Autodesk Inventor part; units mm, degrees
(part 2 of 2)
sketch "Sketch4" plane through (0, 0, 0.5) normal (0, 0, 1) x (1, 0, 0)
  line L0 (210, -1.9975) -> (0, -1.9975) projected
  line L1 (1.9975, -19.0025) -> (23.0025, -19.0025)
  line L2 (23.0025, -19.0025) -> (23.0025, -1.9975)
  line L3 (23.0025, -1.9975) -> (1.9975, -1.9975)
  line L4 (1.9975, -1.9975) -> (1.9975, -19.0025)
  line L5 (34.9975, -1.9975) -> (152.0025, -1.9975)
  line L6 (152.0025, -1.9975) -> (152.0025, -19.0025)
  line L7 (152.0025, -19.0025) -> (34.9975, -19.0025)
  line L8 (34.9975, -19.0025) -> (34.9975, -1.9975)
  line L9 (210, -24.25) -> (210, -1.9975) projected
  line L10 (163.4975, -1.9975) -> (210, -1.9975)
  line L11 (210, -1.9975) -> (210, -19.0025)
  line L12 (210, -19.0025) -> (163.4975, -19.0025)
  line L13 (163.4975, -19.0025) -> (163.4975, -1.9975)
  line L14 (200.5, -48.05) -> (200.5, -24.25) projected
  line L15 (200.5, -29.4975) -> (0, -29.4975)
  line L16 (0, -29.4975) -> (0, -122.9025)
  line L17 (0, -122.9025) -> (216.3009, -122.9025) projected
  line L18 (0, -122.9025) -> (216.3009, -122.9025)
  line L19 (216.3009, -122.9025) -> (216.3009, -105.3171)
  line L20 (216.3009, -103.8025) -> (205.25, -103.8025) projected
  line L21 (216.3009, -105.3171) -> (216.3009, -103.8025)
  line L22 (216.3009, -103.8025) -> (205.25, -103.8025)
  line L23 (200.5, -29.4975) -> (200.5, -48.05)
  line L24 (210.25, -67.15) -> (210.25, -48.05) projected
  line L25 (200.5, -48.05) -> (210.25, -48.05)
  line L26 (215, -67.15) -> (210.25, -67.15) projected
  line L27 (210.25, -48.05) -> (210.25, -67.15)
  line L28 (215, -86.25) -> (215, -67.15) projected
  line L29 (210.25, -67.15) -> (215, -67.15)
  line L30 (215, -67.15) -> (215, -86.25)
  line L31 (205.25, -103.8025) -> (205.25, -86.25) projected
  line L32 (215, -86.25) -> (205.25, -86.25)
  line L33 (205.25, -86.25) -> (205.25, -103.8025)
  line L34 (205.25, -103.8025) -> (216.3009, -103.8025)
  line L35 (163.4975, -1.9975) -> (210, -1.9975)
  line L36 (210, -1.9975) -> (210, -19.0025)
  line L37 (152.0025, -1.9975) -> (34.9975, -1.9975)
  line L38 (23.0025, -1.9975) -> (1.9975, -1.9975)
  line L39 (216.3009, -103.8025) -> (205.25, -103.8025) projected
  line L40 (205.25, -103.8025) -> (205.25, -86.25) projected
  line L41 (205.25, -86.25) -> (215, -86.25) projected
  line L42 (215, -86.25) -> (215, -67.15) projected
  line L43 (215, -67.15) -> (210.25, -67.15) projected
  line L44 (210.25, -67.15) -> (210.25, -48.05) projected
  line L45 (210.25, -48.05) -> (200.5, -48.05) projected
  line L46 (200.5, -48.05) -> (200.5, -24.25) projected
  line L47 (200.5, -24.25) -> (210, -24.25) projected
  line L48 (210, -24.25) -> (210, -1.9975) projected
  line L49 (210, -1.9975) -> (0, -1.9975) projected
  line L50 (0, -1.9975) -> (0, -122.9025) projected
  line L51 (0, -122.9025) -> (216.3009, -122.9025) projected
  line L52 (216.3009, -122.9025) -> (216.3009, -103.8025) projected
  line L53 (119.75, -21.25) -> (163.5, -21.25) projected
  line L54 (163.5, -21.25) -> (163.5, -28.75) projected
  line L55 (163.5, -28.75) -> (119.75, -28.75) projected
  line L56 (119.75, -28.75) -> (119.75, -21.25) projected
  line L57 (67.1017, -107.9725) -> (73.1018, -107.9725) projected
  line L58 (73.1018, -107.9725) -> (73.1018, -120.1725) projected
  line L59 (73.1018, -120.1725) -> (67.1017, -120.1725) projected
  line L60 (67.1017, -120.1725) -> (67.1017, -107.9725) projected
  line L61 (200.6018, -107.9725) -> (206.6018, -107.9725) projected
  line L62 (206.6018, -107.9725) -> (206.6018, -120.1725) projected
  line L63 (206.6018, -120.1725) -> (200.6018, -120.1725) projected
  line L64 (200.6018, -120.1725) -> (200.6018, -107.9725) projected
  line L65 (29, -50.5975) -> (35, -50.5975) projected
  line L66 (35, -50.5975) -> (35, -62.7975) projected
  line L67 (35, -62.7975) -> (29, -62.7975) projected
  line L68 (29, -62.7975) -> (29, -50.5975) projected
  line L69 (5, -50.5975) -> (11, -50.5975) projected
  line L70 (11, -50.5975) -> (11, -62.7975) projected
  line L71 (11, -62.7975) -> (5, -62.7975) projected
  line L72 (5, -62.7975) -> (5, -50.5975) projected
  line L73 (40.4975, -107.8975) -> (54.5025, -107.8975) projected
  line L74 (54.5025, -107.8975) -> (54.5025, -121.9025) projected
  line L75 (54.5025, -121.9025) -> (40.4975, -121.9025) projected
  line L76 (40.4975, -121.9025) -> (40.4975, -107.8975) projected
  line L77 (15.9975, -107.8975) -> (30.0025, -107.8975) projected
  line L78 (30.0025, -107.8975) -> (30.0025, -121.9025) projected
  line L79 (30.0025, -121.9025) -> (15.9975, -121.9025) projected
  line L80 (15.9975, -121.9025) -> (15.9975, -107.8975) projected
  line L81 (188.7475, -88.7975) -> (202.7525, -88.7975) projected
  line L82 (202.7525, -88.7975) -> (202.7525, -102.8025) projected
  line L83 (202.7525, -102.8025) -> (188.7475, -102.8025) projected
  line L84 (188.7475, -102.8025) -> (188.7475, -88.7975) projected
  line L85 (169.7475, -88.7975) -> (183.7525, -88.7975) projected
  line L86 (183.7525, -88.7975) -> (183.7525, -102.8025) projected
  line L87 (183.7525, -102.8025) -> (169.7475, -102.8025) projected
  line L88 (169.7475, -102.8025) -> (169.7475, -88.7975) projected
  line L89 (150.7475, -88.7975) -> (164.7525, -88.7975) projected
  line L90 (164.7525, -88.7975) -> (164.7525, -102.8025) projected
  line L91 (164.7525, -102.8025) -> (150.7475, -102.8025) projected
  line L92 (150.7475, -102.8025) -> (150.7475, -88.7975) projected
  line L93 (131.7475, -88.7975) -> (145.7525, -88.7975) projected
  line L94 (145.7525, -88.7975) -> (145.7525, -102.8025) projected
  line L95 (145.7525, -102.8025) -> (131.7475, -102.8025) projected
  line L96 (131.7475, -102.8025) -> (131.7475, -88.7975) projected
  line L97 (112.7475, -88.7975) -> (126.7525, -88.7975) projected
  line L98 (126.7525, -88.7975) -> (126.7525, -102.8025) projected
  line L99 (126.7525, -102.8025) -> (112.7475, -102.8025) projected
  line L100 (112.7475, -102.8025) -> (112.7475, -88.7975) projected
  line L101 (93.7475, -88.7975) -> (107.7525, -88.7975) projected
  line L102 (107.7525, -88.7975) -> (107.7525, -102.8025) projected
  line L103 (107.7525, -102.8025) -> (93.7475, -102.8025) projected
  line L104 (93.7475, -102.8025) -> (93.7475, -88.7975) projected
  line L105 (74.7475, -88.7975) -> (88.7525, -88.7975) projected
  line L106 (88.7525, -88.7975) -> (88.7525, -102.8025) projected
  line L107 (88.7525, -102.8025) -> (74.7475, -102.8025) projected
  line L108 (74.7475, -102.8025) -> (74.7475, -88.7975) projected
  line L109 (55.7475, -88.7975) -> (69.7525, -88.7975) projected
  line L110 (69.7525, -88.7975) -> (69.7525, -102.8025) projected
  line L111 (69.7525, -102.8025) -> (55.7475, -102.8025) projected
  line L112 (55.7475, -102.8025) -> (55.7475, -88.7975) projected
  line L113 (36.7475, -88.7975) -> (50.7525, -88.7975) projected
  line L114 (50.7525, -88.7975) -> (50.7525, -102.8025) projected
  line L115 (50.7525, -102.8025) -> (36.7475, -102.8025) projected
  line L116 (36.7475, -102.8025) -> (36.7475, -88.7975) projected
  line L117 (10.4975, -88.7975) -> (24.5025, -88.7975) projected
  line L118 (24.5025, -88.7975) -> (24.5025, -102.8025) projected
  line L119 (24.5025, -102.8025) -> (10.4975, -102.8025) projected
  line L120 (10.4975, -102.8025) -> (10.4975, -88.7975) projected
  line L121 (5.9975, -69.6975) -> (20.0025, -69.6975) projected
  line L122 (20.0025, -69.6975) -> (20.0025, -83.7025) projected
  line L123 (20.0025, -83.7025) -> (5.9975, -83.7025) projected
  line L124 (5.9975, -83.7025) -> (5.9975, -69.6975) projected
  line L125 (27.4975, -69.6975) -> (41.5025, -69.6975) projected
  line L126 (41.5025, -69.6975) -> (41.5025, -83.7025) projected
  line L127 (41.5025, -83.7025) -> (27.4975, -83.7025) projected
  line L128 (27.4975, -83.7025) -> (27.4975, -69.6975) projected
  line L129 (46.4975, -69.6975) -> (60.5025, -69.6975) projected
  line L130 (60.5025, -69.6975) -> (60.5025, -83.7025) projected
  line L131 (60.5025, -83.7025) -> (46.4975, -83.7025) projected
  line L132 (46.4975, -83.7025) -> (46.4975, -69.6975) projected
  line L133 (65.4975, -69.6975) -> (79.5025, -69.6975) projected
  line L134 (79.5025, -69.6975) -> (79.5025, -83.7025) projected
  line L135 (79.5025, -83.7025) -> (65.4975, -83.7025) projected
  line L136 (65.4975, -83.7025) -> (65.4975, -69.6975) projected
  line L137 (84.4975, -69.6975) -> (98.5025, -69.6975) projected
  line L138 (98.5025, -69.6975) -> (98.5025, -83.7025) projected
  line L139 (98.5025, -83.7025) -> (84.4975, -83.7025) projected
  line L140 (84.4975, -83.7025) -> (84.4975, -69.6975) projected
  line L141 (103.4975, -69.6975) -> (117.5025, -69.6975) projected
  line L142 (117.5025, -69.6975) -> (117.5025, -83.7025) projected
  line L143 (117.5025, -83.7025) -> (103.4975, -83.7025) projected
  line L144 (103.4975, -83.7025) -> (103.4975, -69.6975) projected
  line L145 (122.4975, -69.6975) -> (136.5025, -69.6975) projected
  line L146 (136.5025, -69.6975) -> (136.5025, -83.7025) projected
  line L147 (136.5025, -83.7025) -> (122.4975, -83.7025) projected
  line L148 (122.4975, -83.7025) -> (122.4975, -69.6975) projected
  line L149 (141.4975, -69.6975) -> (155.5025, -69.6975) projected
  line L150 (155.5025, -69.6975) -> (155.5025, -83.7025) projected
  line L151 (155.5025, -83.7025) -> (141.4975, -83.7025) projected
  line L152 (141.4975, -83.7025) -> (141.4975, -69.6975) projected
  line L153 (160.4975, -69.6975) -> (174.5025, -69.6975) projected
  line L154 (174.5025, -69.6975) -> (174.5025, -83.7025) projected
  line L155 (174.5025, -83.7025) -> (160.4975, -83.7025) projected
  line L156 (160.4975, -83.7025) -> (160.4975, -69.6975) projected
  line L157 (179.4975, -69.6975) -> (193.5025, -69.6975) projected
  line L158 (193.5025, -69.6975) -> (193.5025, -83.7025) projected
  line L159 (193.5025, -83.7025) -> (179.4975, -83.7025) projected
  line L160 (179.4975, -83.7025) -> (179.4975, -69.6975) projected
  line L161 (198.4975, -69.6975) -> (212.5025, -69.6975) projected
  line L162 (212.5025, -69.6975) -> (212.5025, -83.7025) projected
  line L163 (212.5025, -83.7025) -> (198.4975, -83.7025) projected
  line L164 (198.4975, -83.7025) -> (198.4975, -69.6975) projected
  line L165 (193.7475, -50.5975) -> (207.7525, -50.5975) projected
  line L166 (207.7525, -50.5975) -> (207.7525, -64.6025) projected
  line L167 (207.7525, -64.6025) -> (193.7475, -64.6025) projected
  line L168 (193.7475, -64.6025) -> (193.7475, -50.5975) projected
  line L169 (174.7475, -50.5975) -> (188.7525, -50.5975) projected
  line L170 (188.7525, -50.5975) -> (188.7525, -64.6025) projected
  line L171 (188.7525, -64.6025) -> (174.7475, -64.6025) projected
  line L172 (174.7475, -64.6025) -> (174.7475, -50.5975) projected
  line L173 (155.7475, -50.5975) -> (169.7525, -50.5975) projected
  line L174 (169.7525, -50.5975) -> (169.7525, -64.6025) projected
  line L175 (169.7525, -64.6025) -> (155.7475, -64.6025) projected
  line L176 (155.7475, -64.6025) -> (155.7475, -50.5975) projected
  line L177 (136.7475, -50.5975) -> (150.7525, -50.5975) projected
  line L178 (150.7525, -50.5975) -> (150.7525, -64.6025) projected
  line L179 (150.7525, -64.6025) -> (136.7475, -64.6025) projected
  line L180 (136.7475, -64.6025) -> (136.7475, -50.5975) projected
  line L181 (117.7475, -50.5975) -> (131.7525, -50.5975) projected
  line L182 (131.7525, -50.5975) -> (131.7525, -64.6025) projected
  line L183 (131.7525, -64.6025) -> (117.7475, -64.6025) projected
  line L184 (117.7475, -64.6025) -> (117.7475, -50.5975) projected
  line L185 (98.7475, -50.5975) -> (112.7525, -50.5975) projected
  line L186 (112.7525, -50.5975) -> (112.7525, -64.6025) projected
  line L187 (112.7525, -64.6025) -> (98.7475, -64.6025) projected
  line L188 (98.7475, -64.6025) -> (98.7475, -50.5975) projected
  line L189 (79.7475, -50.5975) -> (93.7525, -50.5975) projected
  line L190 (93.7525, -50.5975) -> (93.7525, -64.6025) projected
  line L191 (93.7525, -64.6025) -> (79.7475, -64.6025) projected
  line L192 (79.7475, -64.6025) -> (79.7475, -50.5975) projected
  line L193 (60.7475, -50.5975) -> (74.7525, -50.5975) projected
  line L194 (74.7525, -50.5975) -> (74.7525, -64.6025) projected
  line L195 (74.7525, -64.6025) -> (60.7475, -64.6025) projected
  line L196 (60.7475, -64.6025) -> (60.7475, -50.5975) projected
  line L197 (41.7475, -50.5975) -> (55.7525, -50.5975) projected
  line L198 (55.7525, -50.5975) -> (55.7525, -64.6025) projected
  line L199 (55.7525, -64.6025) -> (41.7475, -64.6025) projected
  line L200 (41.7475, -64.6025) -> (41.7475, -50.5975) projected
  line L201 (12.9975, -50.5975) -> (27.0025, -50.5975) projected
  line L202 (27.0025, -50.5975) -> (27.0025, -64.6025) projected
  line L203 (27.0025, -64.6025) -> (12.9975, -64.6025) projected
  line L204 (12.9975, -64.6025) -> (12.9975, -50.5975) projected
  line L205 (183.9975, -31.4975) -> (198.0025, -31.4975) projected
  line L206 (198.0025, -31.4975) -> (198.0025, -45.5025) projected
  line L207 (198.0025, -45.5025) -> (183.9975, -45.5025) projected
  line L208 (183.9975, -45.5025) -> (183.9975, -31.4975) projected
  line L209 (164.9975, -31.4975) -> (179.0025, -31.4975) projected
  line L210 (179.0025, -31.4975) -> (179.0025, -45.5025) projected
  line L211 (179.0025, -45.5025) -> (164.9975, -45.5025) projected
  line L212 (164.9975, -45.5025) -> (164.9975, -31.4975) projected
  line L213 (145.9975, -31.4975) -> (160.0025, -31.4975) projected
  line L214 (160.0025, -31.4975) -> (160.0025, -45.5025) projected
  line L215 (160.0025, -45.5025) -> (145.9975, -45.5025) projected
  line L216 (145.9975, -45.5025) -> (145.9975, -31.4975) projected
  line L217 (126.9975, -31.4975) -> (141.0025, -31.4975) projected
  line L218 (141.0025, -31.4975) -> (141.0025, -45.5025) projected
  line L219 (141.0025, -45.5025) -> (126.9975, -45.5025) projected
  line L220 (126.9975, -45.5025) -> (126.9975, -31.4975) projected
  line L221 (107.9975, -31.4975) -> (122.0025, -31.4975) projected
  line L222 (122.0025, -31.4975) -> (122.0025, -45.5025) projected
  line L223 (122.0025, -45.5025) -> (107.9975, -45.5025) projected
  line L224 (107.9975, -45.5025) -> (107.9975, -31.4975) projected
  line L225 (88.9975, -31.4975) -> (103.0025, -31.4975) projected
  line L226 (103.0025, -31.4975) -> (103.0025, -45.5025) projected
  line L227 (103.0025, -45.5025) -> (88.9975, -45.5025) projected
  line L228 (88.9975, -45.5025) -> (88.9975, -31.4975) projected
  line L229 (69.9975, -31.4975) -> (84.0025, -31.4975) projected
  line L230 (84.0025, -31.4975) -> (84.0025, -45.5025) projected
  line L231 (84.0025, -45.5025) -> (69.9975, -45.5025) projected
  line L232 (69.9975, -45.5025) -> (69.9975, -31.4975) projected
  line L233 (50.9975, -31.4975) -> (65.0025, -31.4975) projected
  line L234 (65.0025, -31.4975) -> (65.0025, -45.5025) projected
  line L235 (65.0025, -45.5025) -> (50.9975, -45.5025) projected
  line L236 (50.9975, -45.5025) -> (50.9975, -31.4975) projected
  line L237 (31.9975, -31.4975) -> (46.0025, -31.4975) projected
  line L238 (46.0025, -31.4975) -> (46.0025, -45.5025) projected
  line L239 (46.0025, -45.5025) -> (31.9975, -45.5025) projected
  line L240 (31.9975, -45.5025) -> (31.9975, -31.4975) projected
  line L241 (7.9975, -31.4975) -> (22.0025, -31.4975) projected
  line L242 (22.0025, -31.4975) -> (22.0025, -45.5025) projected
  line L243 (22.0025, -45.5025) -> (7.9975, -45.5025) projected
  line L244 (7.9975, -45.5025) -> (7.9975, -31.4975) projected
  line L245 (190.9975, -2.9975) -> (205.0025, -2.9975) projected
  line L246 (205.0025, -2.9975) -> (205.0025, -17.0025) projected
  line L247 (205.0025, -17.0025) -> (190.9975, -17.0025) projected
  line L248 (190.9975, -17.0025) -> (190.9975, -2.9975) projected
  line L249 (166.9975, -2.9975) -> (181.0025, -2.9975) projected
  line L250 (181.0025, -2.9975) -> (181.0025, -17.0025) projected
  line L251 (181.0025, -17.0025) -> (166.9975, -17.0025) projected
  line L252 (166.9975, -17.0025) -> (166.9975, -2.9975) projected
  line L253 (134.4975, -2.9975) -> (148.5025, -2.9975) projected
  line L254 (148.5025, -2.9975) -> (148.5025, -17.0025) projected
  line L255 (148.5025, -17.0025) -> (134.4975, -17.0025) projected
  line L256 (134.4975, -17.0025) -> (134.4975, -2.9975) projected
  line L257 (110.4975, -2.9975) -> (124.5025, -2.9975) projected
  line L258 (124.5025, -2.9975) -> (124.5025, -17.0025) projected
  line L259 (124.5025, -17.0025) -> (110.4975, -17.0025) projected
  line L260 (110.4975, -17.0025) -> (110.4975, -2.9975) projected
  line L261 (86.4975, -2.9975) -> (100.5025, -2.9975) projected
  line L262 (100.5025, -2.9975) -> (100.5025, -17.0025) projected
  line L263 (100.5025, -17.0025) -> (86.4975, -17.0025) projected
  line L264 (86.4975, -17.0025) -> (86.4975, -2.9975) projected
  line L265 (62.4975, -2.9975) -> (76.5025, -2.9975) projected
  line L266 (76.5025, -2.9975) -> (76.5025, -17.0025) projected
  line L267 (76.5025, -17.0025) -> (62.4975, -17.0025) projected
  line L268 (62.4975, -17.0025) -> (62.4975, -2.9975) projected
  line L269 (38.4975, -2.9975) -> (52.5025, -2.9975) projected
  line L270 (52.5025, -2.9975) -> (52.5025, -17.0025) projected
  line L271 (52.5025, -17.0025) -> (38.4975, -17.0025) projected
  line L272 (38.4975, -17.0025) -> (38.4975, -2.9975) projected
  line L273 (5.4975, -2.9975) -> (19.5025, -2.9975) projected
  line L274 (19.5025, -2.9975) -> (19.5025, -17.0025) projected
  line L275 (19.5025, -17.0025) -> (5.4975, -17.0025) projected
  line L276 (5.4975, -17.0025) -> (5.4975, -2.9975) projected
  line L277 (129.8493, -107.9725) -> (143.8543, -107.9725) projected
  line L278 (143.8543, -107.9725) -> (143.8543, -121.9775) projected
  line L279 (143.8543, -121.9775) -> (129.8493, -121.9775) projected
  line L280 (129.8493, -121.9775) -> (129.8493, -107.9725) projected
  line L281 (0, -1.9975) -> (0, -122.9025) projected
  line L282 (0, -103.9025) -> (11, -103.9025)
  line L283 (11, -103.9025) -> (11, -122.9025)
  point P0 (0, 0)
  point P1 (5.4975, -10)
  point P2 (1.9975, -1.9975)
  dimension "d124" = 19
  dimension "d125" = 11
  dimension "d126" = 2
  dimension "d127" = 2
  dimension "d128" = 3.5
  dimension "d129" = 3.5
  dimension "d130" = 3.5
  dimension "d131" = 3.5
  dimension "d132" = 3.5
  constraints: 64 end point, 14 perpendicular, 10 collinear, 9 point on line, 6 parallel, 3 horizontal, 1 midpoint, 1 vertical
  measures "d124" distance of L282.end L283.end
  measures "d125" distance of L282.start L282.end
  measures "d126" distance between parallel lines of L15 L241
  measures "d127" distance between parallel lines of L275 L1
  measures "d128" distance from line of point (5.497, -10) L4
  measures "d129" distance between parallel lines of L2 L274
  measures "d130" distance between parallel lines of L272 L8
  measures "d131" distance between parallel lines of L6 L254
  measures "d132" distance between parallel lines of L252 L13
extrude "Extrusion2" add sketch "Sketch4" along normal blind 2.5 contours L9 L12 L13 L0 | L6 L7 L8 L0 | L2 L1 L4 L0 | L14 L25 L24 L26 L28 L32 L31 L20 L21 L19 L17 L283 L282 L16 L15 | L282 L283 L17 L16
sketch "Sketch5" plane through (0, 0, 0) normal (0, 0, -1) x (-1, 0, 0)
  line L0 (-200.6018, -107.9725) -> (-206.6018, -107.9725) construction
  line L1 (-206.6018, -107.9725) -> (-206.6018, -120.1725) construction
  line L2 (-200.6018, -120.1725) -> (-200.6018, -107.9725) construction
  line L3 (-206.6018, -120.1725) -> (-200.6018, -120.1725) construction
  line L4 (-67.1018, -107.9725) -> (-73.1017, -107.9725) construction
  line L5 (-67.1018, -120.1725) -> (-67.1018, -107.9725) construction
  line L6 (-73.1017, -107.9725) -> (-73.1018, -120.1725) construction
  line L7 (-73.1018, -120.1725) -> (-67.1018, -120.1725) construction
  line L8 (-5, -50.5975) -> (-11, -50.5975) construction
  line L9 (-5, -62.7975) -> (-5, -50.5975) construction
  line L10 (-11, -62.7975) -> (-5, -62.7975) construction
  line L11 (-11, -50.5975) -> (-11, -62.7975) construction
  line L12 (-29, -50.5975) -> (-35, -50.5975) construction
  line L13 (-29, -62.7975) -> (-29, -50.5975) construction
  line L14 (-35, -50.5975) -> (-35, -62.7975) construction
  line L15 (-35, -62.7975) -> (-29, -62.7975) construction
  line L16 (-35, -47.5975) -> (-5, -47.5975)
  line L17 (-5, -47.5975) -> (-5, -64.7975)
  line L18 (-5, -64.7975) -> (-11, -64.7975)
  line L19 (-11, -64.7975) -> (-11, -54.5975)
  line L20 (-11, -54.5975) -> (-29, -54.5975)
  line L21 (-29, -64.7975) -> (-29, -54.5975)
  line L22 (-29, -64.7975) -> (-35, -64.7975)
  line L23 (-35, -64.7975) -> (-35, -47.5975)
  line L24 (-206.6018, -122.1725) -> (-206.6018, -104.9725)
  line L25 (-206.6018, -104.9725) -> (-67.1018, -104.9725)
  line L26 (-67.1018, -104.9725) -> (-67.1018, -122.1725)
  line L27 (0, -122.9025) -> (-216.3009, -122.9025) projected
  line L28 (-67.1018, -122.1725) -> (-73.1017, -122.1725)
  line L29 (-73.1017, -122.1725) -> (-73.1017, -111.9725)
  line L30 (-200.6018, -111.9725) -> (-73.1017, -111.9725)
  line L31 (-200.6018, -111.9725) -> (-200.6018, -122.1725)
  line L32 (-206.6018, -122.1725) -> (-200.6018, -122.1725)
  point P0 (0, 0)
  point P1 (-11, -122.9025)
  dimension "d135" = 3
  dimension "d136" = 2
  dimension "d137" = 4
  dimension "d138" = 2
  dimension "d139" = 3
  dimension "d140" = 4
  constraints: 32 end point, 11 point on line, 7 perpendicular, 4 collinear, 1 horizontal
  measures "d135" distance between parallel lines of L16 L12
  measures "d136" distance between parallel lines of L22 L15
  measures "d137" distance between parallel lines of L20 L12
  measures "d138" distance between parallel lines of L32 L3
  measures "d139" distance between parallel lines of L0 L25
  measures "d140" distance between parallel lines of L30 L0
extrude "Extrusion3" cut sketch "Sketch5" against normal blind 2
equation "\"d0\" = sw"
equation "\"d1\" = sw"
equation "\"d3\" = sw"
equation "\"d4\" = sw"
equation "\"d5\" = sw"
equation "\"d6\" = sw"
equation "\"d7\" = sw"
equation "\"d8\" = sw"
equation "\"d9\" = sw"
equation "\"d10\" = sw"
equation "\"d11\" = sw"
equation "\"d12\" = sw"
equation "\"d13\" = sw"
equation "\"d14\" = sw"
equation "\"d15\" = sw"
equation "\"d16\" = sw"
equation "\"d17\" = sw"
equation "\"d18\" = sw"
equation "\"d19\" = sw"
equation "\"d20\" = sw"
equation "\"d21\" = sw"
equation "\"d22\" = sw"
equation "\"d23\" = sw"
equation "\"d24\" = sw"
equation "\"d25\" = sw"
equation "\"d26\" = sw"
equation "\"d27\" = sw"
equation "\"d28\" = sw"
equation "\"d29\" = sw"
equation "\"d30\" = sw"
equation "\"d31\" = sw"
equation "\"d32\" = sw"
equation "\"d33\" = sw"
equation "\"d34\" = sw"
equation "\"d35\" = sw"
equation "\"d36\" = sw"
equation "\"d37\" = sw"
equation "\"d38\" = sw"
equation "\"d39\" = sw"
equation "\"d40\" = sw"
equation "\"d41\" = sw"
equation "\"d42\" = sw"
equation "\"d43\" = sw"
equation "\"d44\" = sw"
equation "\"d45\" = sw"
equation "\"d46\" = sw"
equation "\"d47\" = sw"
equation "\"d48\" = sw"
equation "\"d49\" = sw"
equation "\"d50\" = sw"
equation "\"d51\" = sw"
equation "\"d52\" = sw"
equation "\"d53\" = sw"
equation "\"d54\" = sw"
equation "\"d55\" = sw"
equation "\"d56\" = sw"
equation "\"d57\" = sw"
equation "\"d58\" = sw"
equation "\"d59\" = sw"
equation "\"d60\" = sw"
equation "\"d61\" = sw"
equation "\"d62\" = sw"
equation "\"d63\" = sw"
equation "\"d64\" = sw"
equation "\"d127\" = d126"
equation "\"d129\" = d128"
equation "\"d130\" = d128"
equation "\"d131\" = d128"
equation "\"d132\" = d128"
equation "\"sw\" = 14.005"
body "Solid1"
